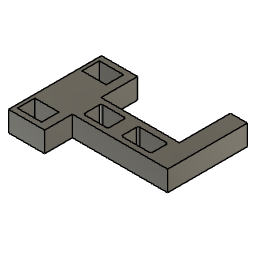
battery_fixture_typeC v3 (Autodesk Fusion 360 design; units mm, degrees)
Autodesk Fusion 360 part; units mm, degrees
sketch "スケッチ1" plane through (0, 0, 0) normal (0, 0, 1) x (1, 0, 0)
  line L0 (3.2, 13.7) -> (17.7, 13.7)
  line L1 (17.7, 13.7) -> (17.7, 3.2)
  line L2 (17.7, 3.2) -> (3.2, 3.2)
  line L3 (3.2, 3.2) -> (3.2, 13.7)
  line L4 (25.5, 13.2) -> (43, 13.2)
  line L5 (43, 13.2) -> (43, 3.2)
  line L6 (43, 3.2) -> (25.5, 3.2)
  line L7 (25.5, 3.2) -> (25.5, 13.2)
  line L8 (0, 0) -> (46, 0)
  line L9 (46, 0) -> (46, 16.9)
  line L10 (46, 16.9) -> (0, 16.9)
  line L11 (0, 16.9) -> (0, 0)
  line L12 (46, 0) -> (56, 0)
  line L13 (56, 0) -> (56, 46.9)
  line L14 (56, 46.9) -> (46, 46.9)
  line L15 (46, 46.9) -> (46, 0)
  line L16 (-19.2, 35.1) -> (-5, 35.1)
  line L17 (-5, 35.1) -> (-5, 24.9)
  line L18 (-5, 24.9) -> (-19.2, 24.9)
  line L19 (-19.2, 24.9) -> (-19.2, 35.1)
  line L20 (-19.2, -2.9) -> (-5, -2.9)
  line L21 (-5, -2.9) -> (-5, -13.1)
  line L22 (-5, -13.1) -> (-19.2, -13.1)
  line L23 (-19.2, -13.1) -> (-19.2, -2.9)
  line L24 (0, 16.9) -> (0, 38.3)
  line L25 (0, 38.3) -> (-21.2, 38.3)
  line L26 (-21.2, 38.3) -> (-21.2, -16.3)
  line L27 (-21.2, -16.3) -> (0, -16.3)
  line L28 (0, -16.3) -> (0, 0)
  dimension "d1" = 10.5
  dimension "d2" = 10
  dimension "d3" = 14.5
  dimension "d4" = 17.5
  dimension "d5" = 7.8
  dimension "d6" = 3.2
  dimension "d7" = 3.2
  dimension "d8" = 3.2
  dimension "d9" = 3.2
  dimension "d10" = 46
  dimension "d11" = 10
  dimension "d12" = 30
  dimension "d17" = 14.2
  dimension "d18" = 14.2
  dimension "d19" = 10.2
  dimension "d20" = 10.2
  dimension "d21" = 27.8
  dimension "d22" = 8
  dimension "d23" = 5
  dimension "d24" = 5
  dimension "d25" = 2
  dimension "d26" = 3.2
  dimension "d27" = 3.2
  constraint horizontal L0
  constraint vertical L1
  constraint horizontal L2
  constraint vertical L3
  constraint horizontal L4
  constraint vertical L5
  constraint horizontal L6
  constraint vertical L7
  constraint horizontal L8
  constraint vertical L9
  constraint horizontal L10
  constraint vertical L11
  constraint coincident L8.start L11.end
  constraint horizontal L12
  constraint vertical L13
  constraint horizontal L14
  constraint vertical L15
  constraint horizontal L16
  constraint vertical L17
  constraint horizontal L18
  constraint vertical L19
  constraint horizontal L20
  constraint vertical L21
  constraint horizontal L22
  constraint vertical L23
  constraint perpendicular L10 L24
  constraint perpendicular L24 L25
  constraint perpendicular L25 L26
  constraint perpendicular L11 L27
  constraint perpendicular L8 L28
  measures "d1" distance of L0.start L2.end
  measures "d2" distance of L4.end L5.end
  measures "d3" distance of L1.end L2.end
  measures "d4" distance of L5.end L6.end
  measures "d5" distance of L1 L7
  measures "d6" distance of L2 L8
  measures "d7" distance of L8.start L3
  measures "d8" distance of L0 L10
  measures "d9" distance of L8.start L6
  measures "d10" distance of L8.start L8.end
  measures "d11" distance of L8.end L12.end
  measures "d12" distance of L10 L14
  measures "d17" distance of L16.start L16.end
  measures "d18" distance of L21.end L22.end
  measures "d19" distance of L16.start L18.end
  measures "d20" distance of L20.start L22.end
  measures "d21" distance of L18 L20
  measures "d22" distance of L10 L18
  measures "d23" distance of L8.start L17
  measures "d24" distance of L8.start L21
  measures "d25" distance of L19 L26
  measures "d26" distance of L16 L25
  measures "d27" distance of L22 L27
extrude "押し出し1" add sketch "スケッチ1" along normal blind 12
fillet "フィレット1" radius 1 8 edges at (3.2, 13.7, 6) (25.5, 13.2, 6) (3.2, 3.2, 6) (25.5, 3.2, 6) (43, 3.2, 6) (17.7, 3.2, 6) (43, 13.2, 6) (17.7, 13.7, 6)
